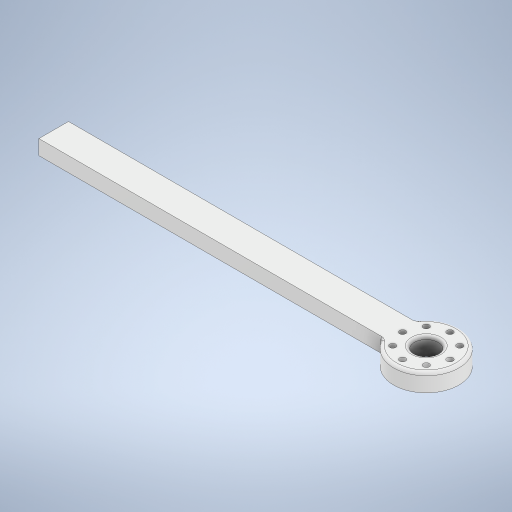
# Autodesk Inventor part: 팔
Saved by Autodesk Inventor 2024.3 (Build 283343000, 343)
## iProperties
Created: 2024-09-10
Part Number: 팔
Material: ABS 플라스틱
Document SubType Name: Modeling
Designer: naru4
Density: 1.06 g/cm^3
Appearance: 매끄러움 - 흰색
Mass: 4.00291 g
Surface Area: 36.2591 cm^2
Volume: 3.77633 cm^3
Author: naru4
Autodesk Inventor part; units mm, degrees
ref_plane "YZ Plane" through (0, 0, 0) normal (1, 0, 0) x (0, 1, 0)
ref_plane "XZ Plane" through (0, 0, 0) normal (0, 1, 0) x (-1, 0, 0)
ref_plane "XY Plane" through (0, 0, 0) normal (0, 0, 1) x (1, 0, 0)
sketch "스케치1" plane through (0, 0, 0) normal (0, 1, 0) x (-1, 0, 0)
  circle A0 centre (-0.1334, 0.1917) radius 4
  circle A1 centre (-0.1334, 0.1917) radius 11
  circle A2 centre (-0.1334, 0.1917) radius 11
  circle A3 centre (-0.1334, 0.1917) radius 8
  circle A4 centre (-0.1334, 8.1917) radius 1
  circle A5 centre (-5.7903, 5.8486) radius 1
  circle A6 centre (-8.1334, 0.1917) radius 1
  circle A7 centre (-5.7903, -5.4651) radius 1
  circle A8 centre (-0.1334, -7.8083) radius 1
  circle A9 centre (5.5235, -5.4651) radius 1
  circle A10 centre (7.8666, 0.1917) radius 1
  circle A11 centre (5.5235, 5.8486) radius 1
  line L0 (0, 0) -> (0, -10.8075)
  line L1 (10.8649, 0) -> (125.8649, 0)
  line L2 (125.8649, 0) -> (125.8649, -5)
  line L3 (125.8649, -5) -> (9.5643, -5)
  line L4 (125.8649, 0) -> (125.8649, 5)
  line L5 (125.8649, 5) -> (9.7601, 5)
  point P0 (9.5643, -5)
  point P1 (9.7601, 5)
  dimension "d2" = 16
  dimension "d3" = 2
  dimension "d4" = 360
  dimension "d5" = 115
  dimension "d6" = 5
  dimension "d7" = 5
  constraints: 12 end point, 11 centre point, 4 point on circle, 3 perpendicular, 1 coincident, 1 horizontal, 1 point on line, 1 vertical, 1 vertical alignment, 22 other
  measures "d3" diameter of A4
  measures "d5" distance of L1.start L1.end
  measures "d6" distance of L1.end L2.end
  measures "d7" distance of L1.end L4.end
extrude "돌출1" add sketch "스케치1" along normal blind 3 contours A1 | A1 L5 L4 L1 | L1 L2 L3 A1 | A10 A3 A9 A8 A7 A6 A5 A4 A11
fillet "모깎기1" radius 1 4 edges at (-9.7601, 1.5, 5) (-9.5643, 1.5, -5) (4.1334, 3, 0.1917) (11.1313, 3, 0.407)
sketch "스케치3" plane through (0, 0, 0) normal (0, -1, 0) x (1, 0, 0)
  arc A0 (-10.3673, 5) -> (-9.4922, 5.516) centre (-10.3673, 6) ccw projected
  arc A1 (-9.2892, -5.484) -> (-9.4922, 5.516) centre (0.1334, 0.1917) ccw projected
  arc A2 (-9.4922, 5.516) -> (-9.2892, -5.484) centre (0.1334, 0.1917) ccw
  arc A3 (-10.3673, 5) -> (-9.4922, 5.516) centre (-10.3673, 6) ccw
  arc A4 (-9.2892, -5.484) -> (-10.1458, -5) centre (-10.1458, -6) ccw projected
  arc A5 (-9.2892, -5.484) -> (-10.1458, -5) centre (-10.1458, -6) ccw
  line L0 (-125.8649, -5) -> (-125.8649, 5) projected
  line L1 (-10.1458, -5) -> (-125.8649, -5)
  line L2 (-125.8649, -5) -> (-125.8649, 5)
  line L3 (-125.8649, 5) -> (-10.3673, 5)
  point P0 (0, 0)
  constraints: 6 end point, 6 point on circle, 3 centre point, 3 tangent, 1 collinear, 1 horizontal, 1 perpendicular
extrude "돌출3" add sketch "스케치3" along normal blind 2 contours A0 A2 A4 L1 L0 L3
thicken "두껍게 하기1" operation add thickness 3 both sides no extend neighbours no toward (0, -1, 0) faces at (3.6327, 0, 8.2973)
sketch "스케치4" plane through (-125.8649, 3, -5) normal (-1, 0, 0) x (0, 0, 1)
  circle A0 centre (5, -3) radius 1.5
  dimension "d20" = 3
  constraints: 1 centre point, 1 coincident
  measures "d20" diameter of A0
extrude "돌출4" cut sketch "스케치4" against normal blind 4
